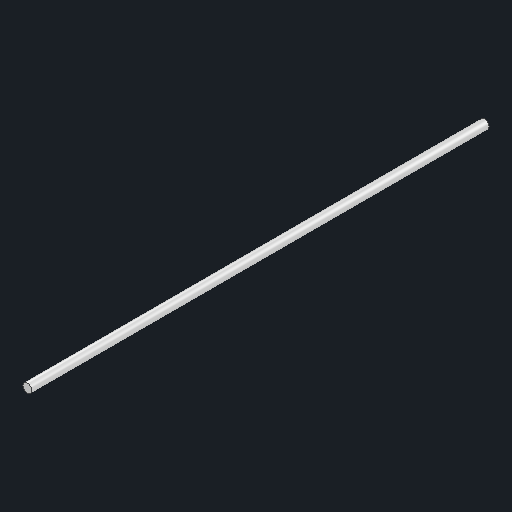
# Autodesk Inventor part: Guide Rod
Saved by Autodesk Inventor 2024.1 (Build 281209000, 209)
## iProperties
Created: 2023-08-04
Part Number: Guide Rod
Material: Stainless Steel
Document SubType Name: Modeling
Designer: jaege
Density: 8 g/cm^3
Appearance: Semi-Polished
Mass: 164.067 g
Surface Area: 103.547 cm^2
Volume: 20.5083 cm^3
Author: jaege
Autodesk Inventor part; units mm, degrees
ref_plane "YZ Plane" through (0, 0, 0) normal (1, 0, 0) x (0, 1, 0)
ref_plane "XZ Plane" through (0, 0, 0) normal (0, 1, 0) x (-1, 0, 0)
sketch "Sketch1" plane through (0, 0, 0) normal (0, 0, 1) x (1, 0, 0)
  circle A0 centre (69.5, 0) radius 4 projected
  point P0 (0, 0)
ref_plane "Work Plane1" through (36.5, 100, 408) normal (0, 0, 1) x (1, 0, 0)
extrude "Extrusion1" add sketch "Sketch1" along normal up to surface (408 mm away)
body "Solid1"
